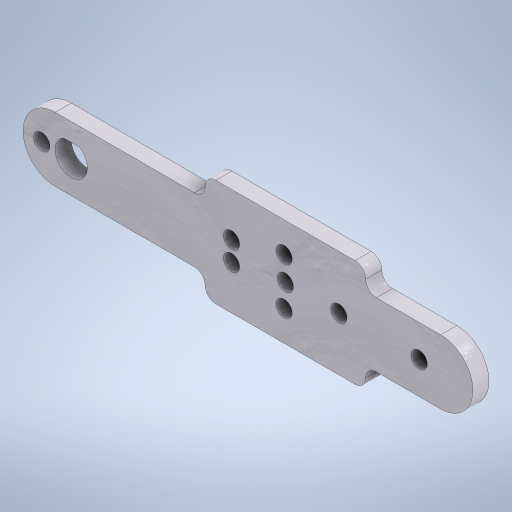
# Autodesk Inventor part: Arm1
Saved by Autodesk Inventor 2023 (Build 270158000, 158)
## iProperties
Created: 2024-02-04
Part Number: Arm1
Material: Aluminum 6061, Welded
Document SubType Name: Modeling
Designer: victo
Density: 2.7 g/cm^3
Appearance: Weld - Aluminum
Author: victo
Autodesk Inventor part; units mm, degrees
ref_plane "YZ Plane" through (0, 0, 0) normal (1, 0, 0) x (0, 1, 0)
ref_plane "XZ Plane" through (0, 0, 0) normal (0, 1, 0) x (-1, 0, 0)
ref_plane "XY Plane" through (0, 0, 0) normal (0, 0, 1) x (1, 0, 0)
sketch "Sketch1" plane through (0, 0, 0) normal (0, 0, 1) x (1, 0, 0)
  circle A0 centre (0, 0) radius 3
  line L0 (-1.4524, 2.625) -> (1.4524, 2.625)
  line L1 (-4.1421, -10) -> (-10, -4.1421)
  line L2 (-10, -4.1421) -> (-10, 4.1421)
  line L3 (-10, 4.1421) -> (-4.1421, 10)
  line L4 (-4.1421, 10) -> (4.1421, 10)
  line L5 (4.1421, 10) -> (10, 4.1421)
  line L6 (10, 4.1421) -> (10, -4.1421)
  line L7 (10, -4.1421) -> (4.1421, -10)
  line L8 (4.1421, -10) -> (-4.1421, -10)
  circle A1 centre (29.944, -1.8315) radius 1.5
  circle A2 centre (29.944, 1.8315) radius 1.5
  circle A3 centre (0, 0) radius 30 construction
  line L9 (0, 0) -> (30, 0) construction
  line L10 (0, 0) -> (29.944, 1.8315) construction
  line L11 (0, 0) -> (29.944, -1.8315) construction
  circle A4 centre (0, 0) radius 40 construction
  circle A5 centre (39.7623, 4.3547) radius 1.5
  circle A6 centre (40, 0) radius 1.5
  circle A7 centre (39.7623, -4.3547) radius 1.5
  line L12 (0, 0) -> (39.7623, 4.3547) construction
  line L13 (40, 0) -> (0, 0) construction
  line L14 (0, 0) -> (39.7623, -4.3547) construction
  circle A8 centre (50, 0) radius 1.5
  circle A9 centre (65, 0) radius 1.5
  circle A10 centre (-5.5, 0) radius 1.5
  line L15 (0, 0) -> (65, 0) construction
  line L16 (0, -10) -> (65, -10)
  line L17 (65, 10) -> (0, 10)
  arc A11 (0, 10) -> (0, -10) centre (0, 0) ccw
  arc A12 (65, -10) -> (65, 10) centre (65, 0) ccw
  line L18 (0, 10) -> (-10, 10)
  line L19 (-10, 10) -> (-10, -10)
  line L20 (-10, -10) -> (0, -10)
  line L21 (0, -10) -> (0, 10)
  line L22 (65, 10) -> (75, 10)
  line L23 (75, 10) -> (75, -10)
  line L24 (75, -10) -> (65, -10)
  line L25 (65, -10) -> (65, 10)
  point P0 (32.5, 0)
  point P1 (4.1421, -10)
  point P2 (0, 10)
  point P3 (0, 0)
  point P4 (65, 0)
  point P5 (75, 0)
  point P6 (-10, 0)
  dimension "d0" = 6
  dimension "d1" = 2.625
  dimension "d2" = 20
  dimension "d3" = 3
  dimension "d4" = 3
  dimension "d5" = 60
  dimension "d6" = 3.5
  dimension "d7" = 3.5
  dimension "d8" = 80
  dimension "d9" = 3
  dimension "d10" = 3
  dimension "d11" = 3
  dimension "d12" = 0
  dimension "d13" = 6.25
  dimension "d14" = 6.25
  dimension "d15" = 3
  dimension "d16" = 3
  dimension "d17" = 0
  dimension "d18" = 50
  dimension "d19" = 0
  dimension "d20" = 65
  dimension "d21" = 3
  dimension "d22" = 0
  dimension "d23" = 5.5
  dimension "d24" = 20
  dimension "d25" = 32.5
  dimension "d36" = 10
  dimension "d37" = 10
  dimension "d38" = 20
  constraints: 54 end point, 13 centre point, 12 point on circle, 5 horizontal, 5 parallel, 4 coincident, 4 tangent, 3 midpoint, 2 perpendicular, 1 collinear, 17 other
  measures "d0" diameter of A0
  measures "d1" distance from line of L0 point (0, 0)
  measures "d2" distance between parallel lines of L4 L8
  measures "d3" diameter of A1
  measures "d4" diameter of A2
  measures "d5" diameter of A3
  measures "d6" angle of L9 L10
  measures "d7" angle of L9 L11
  measures "d8" diameter of A4
  measures "d9" diameter of A5
  measures "d10" diameter of A6
  measures "d11" diameter of A7
  measures "d12" distance between parallel lines of L9 L13
  measures "d13" angle of L9 L12
  measures "d14" angle of L13 L14
  measures "d15" diameter of A8
  measures "d16" diameter of A9
  measures "d17" distance from line of A8.centre L9
  measures "d18" distance of point (0, 0) A8.centre
  measures "d19" vertical distance of point (0, 0) L15.end
  measures "d20" distance of point (0, 0) L15.end
  measures "d21" diameter of A10
  measures "d22" distance from line of A10.centre L9
  measures "d23" distance of point (0, 0) A10.centre
  measures "d24" diameter of A12
  measures "d25" distance of point (32.5, 0) L15.end
  measures "d36" distance from line of point (0, 0) L19
  measures "d37" distance from line of point (65, 0) L23
  measures "d38" distance between parallel lines of L22 L24
extrude "Extrusion1" add sketch "Sketch1" along normal blind 3 contours A0 L21 L4 L5 L6 L7 L8 | L0 L21 A0 | L21 A11 A0 | L21 L0 A0 | L8 L1 A11 | A11 L3 L4 | L7 L6 L5 L17 L25 A9 L16 | L20 L19 L1 | L1 L2 A11 | L3 L19 L18 | A11 L2 L3 | L25 A9 A12 | A12 L23 L24 | L22 L23 A12 picked at (0.8147, 2.6938) picked at (-0.8147, 2.6938)
sketch "Sketch2" plane through (0, 0, 3) normal (0, 0, 1) x (1, 0, 0)
  line L0 (75, 10) -> (-10, 10) projected
  line L1 (-10, -10) -> (75, -10) projected
  line L2 (25, 10) -> (55, 10)
  line L3 (55, 10) -> (55, -10)
  line L4 (55, -10) -> (25, -10)
  line L5 (25, -10) -> (25, 10)
  line L6 (25, 6) -> (-9, 6)
  line L7 (-9, 6) -> (-9, -6)
  line L8 (-9, -6) -> (25, -6)
  line L9 (25, -6) -> (25, 6)
  line L10 (55, 6) -> (75, 6)
  line L11 (75, 6) -> (75, -6)
  line L12 (75, -6) -> (55, -6)
  line L13 (55, -6) -> (55, 6)
  circle A0 centre (65, 0) radius 1.5 projected
  line L14 (75, 10) -> (-10, 10) projected
  line L15 (-10, 10) -> (-10, -10) projected
  line L16 (-10, -10) -> (75, -10) projected
  line L17 (75, -10) -> (75, 10) projected
  arc A1 (-1.4524, 2.625) -> (1.4524, 2.625) centre (0, 0) ccw projected
  circle A2 centre (29.944, -1.8315) radius 1.5 projected
  circle A3 centre (29.944, 1.8315) radius 1.5 projected
  circle A4 centre (39.7623, 4.3547) radius 1.5 projected
  circle A5 centre (40, 0) radius 1.5 projected
  circle A6 centre (39.7623, -4.3547) radius 1.5 projected
  circle A7 centre (50, 0) radius 1.5 projected
  circle A8 centre (65, 0) radius 1.5 projected
  line L18 (-1.4524, 2.625) -> (1.4524, 2.625) projected
  point P0 (-9, 0)
  point P1 (55, -6)
  point P2 (-10, -6)
  point P3 (25, -6)
  point P4 (-10, 6)
  dimension "d28" = 6
  dimension "d29" = 6
  dimension "d30" = 9
  dimension "d31" = 6
  dimension "d32" = 10
  dimension "d33" = 6
  dimension "d34" = 10
  dimension "d39" = 25
  constraints: 24 end point, 6 parallel, 4 point on line, 3 horizontal, 3 perpendicular, 1 midpoint
  measures "d28" distance from line of L6 point (0, 0)
  measures "d29" distance from line of point (0, 0) L8
  measures "d30" distance of point (-9, 0) point (0, 0)
  measures "d31" distance from line of A0.centre L10
  measures "d32" distance from line of A0.centre L11
  measures "d33" distance from line of A0.centre L12
  measures "d34" distance from line of L3 A0.centre
  measures "d39" distance from line of point (0, 0) L5
extrude "Extrusion2" cut sketch "Sketch2" against normal up to surface (3 mm away) contours L17 L10 L3 L0 | L5 L6 L7 L8 L1 L15 L0 | L17 L1 L3 L12
fillet "Fillet1" radius 2 8 edges at (25, -6, 1.5) (25, -10, 1.5) (55, -10, 1.5) (55, -6, 1.5) (25, 10, 1.5) (25, 6, 1.5) (55, 10, 1.5) (55, 6, 1.5)
fillet "Fillet1" radius 6 4 edges at (75, 6, 1.5) (75, -6, 1.5) (-9, 6, 1.5) (-9, -6, 1.5)
equation "\"d7\" = d6"
equation "\"d14\" = d13"
equation "\"d29\" = d28"
equation "\"d31\" = d28"
equation "\"d33\" = d28"
body "Solid1"
